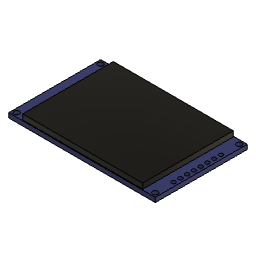
DisplaySquare (Autodesk Fusion 360 design; units mm, degrees)
Autodesk Fusion 360 part; units mm, degrees
sketch "Sketch1" plane through (0, 0, 0) normal (0, 0, 1) x (1, 0, 0)
  line L0 (27.5, -17.25) -> (-27.5, -17.25)
  line L1 (-27.5, -17.25) -> (-27.5, 17.25)
  line L2 (-27.5, 17.25) -> (27.5, 17.25)
  line L3 (27.5, 17.25) -> (27.5, -17.25)
  line L4 (27.5, -17.25) -> (-27.5, 17.25) construction
  line L5 (-27.5, -17.25) -> (27.5, 17.25) construction
  line L6 (22.5, -17) -> (-22.5, -17)
  line L7 (-22.5, -17) -> (-22.5, 17)
  line L8 (-22.5, 17) -> (22.5, 17)
  line L9 (22.5, 17) -> (22.5, -17)
  line L10 (22.5, -17) -> (-22.5, 17) construction
  line L11 (-22.5, -17) -> (22.5, 17) construction
  circle A0 centre (26, 15.75) radius 1
  line L12 (0, 17.25) -> (0, -17.25) construction
  line L13 (27.5, 0) -> (-27.5, 0) construction
  circle A1 centre (-26, 15.75) radius 1
  circle A2 centre (-26, -15.75) radius 1
  circle A3 centre (26, -15.75) radius 1
  circle A4 centre (26, 1.27) radius 0.75
  circle A5 centre (26, 3.81) radius 0.75
  circle A6 centre (26, 6.35) radius 0.75
  circle A7 centre (26, 8.89) radius 0.75
  line L14 (26, 17.25) -> (26, -17.25)
  circle A8 centre (26, -1.27) radius 0.75
  circle A9 centre (26, -3.81) radius 0.75
  circle A10 centre (26, -6.35) radius 0.75
  circle A11 centre (26, -8.89) radius 0.75
  point P0 (25.0526, 0)
  dimension "d29" = 34.5
  dimension "d30" = 55
  dimension "d31" = 45
  dimension "d32" = 34
  dimension "d33" = 2
  dimension "d34" = 1.5
  dimension "d35" = 1.5
  dimension "d37" = 1.5
  dimension "d41" = 0
  dimension "d42" = 2.54
  dimension "d43" = 1.27
  dimension "d44" = 1.5
  constraint horizontal L0
  constraint perpendicular L0 L1
  constraint parallel L0 L2
  constraint parallel L1 L3
  constraint coincident L4 origin
  constraint coincident L5 origin
  constraint horizontal L6
  constraint perpendicular L6 L7
  constraint parallel L6 L8
  constraint parallel L7 L9
  constraint coincident L10 origin
  constraint coincident L11 origin
  constraint midpoint L2 L12.start
  constraint midpoint L0 L12.end
  constraint midpoint L3 L13.start
  constraint midpoint L1 L13.end
  constraint symmetric A0 L12 A1
  constraint symmetric A0 L13 A3
  constraint symmetric L13 A1 A2
  constraint coincident L13 P0
  constraint coincident L2 L14.start
  constraint coincident L0 L14.end
  constraint perpendicular L0 L14
  constraint coincident A4.centre L14
  constraint symmetric L13 A4 A8
  constraint symmetric L13 A5 A9
  constraint symmetric L13 A6 A10
  constraint symmetric L13 A7 A11
  measures "d29" distance of L0.end L1.end
  measures "d30" distance of L1.end L2.end
  measures "d31" distance of L7.end L8.end
  measures "d32" distance of L6.end L7.end
  measures "d33" diameter of A0
  measures "d34" distance of L3 A0.centre
  measures "d35" distance of L2 A0.centre
  measures "d37" diameter of A4
  measures "d43" distance of L13 A4.centre
  measures "d44" distance of L3 L14
extrude "Extrude1" add sketch "Sketch1" along normal blind 1.7 contours L0 L2 L3 A0 A3 A4 A5 A6 A7 L14 A8 A9 A10 A11 | L0 L1 L2 A0 A3 A4 A5 A6 A7 L14 A8 A9 A10 A11 | L6 L7 L8 L9 makes body 1
extrude "Extrude2" add sketch "Sketch1" along normal blind 2 from surface at 1.7 separate body contours L6 L7 L8 L9 makes body 2
equation "d35 = d34"
equation "d37 = d36"
equation "d36 = 1.5 mm"
